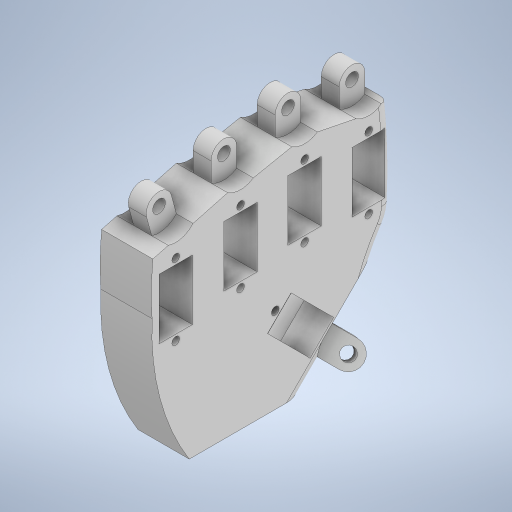
# Autodesk Inventor part: 손바닥
Saved by Autodesk Inventor 2024 (Build 280153000, 153)
## iProperties
Created: 2023-05-04
Part Number: 손바닥
Material: 일반
Document SubType Name: Modeling
Designer: Lenovo
Density: 1 g/cm^3
Appearance: 기본값
Author: Lenovo
Autodesk Inventor part; units mm, degrees
sketch "스케치1" plane through (0, 0, 0) normal (1, 0, 0) x (0, 1, 0)
  circle A0 centre (0, 0) radius 2.5
  arc A1 (0, -5) -> (0, 5) centre (0, 0) ccw
  arc A2 (-7.4833, 5) -> (-7.4833, -5) centre (0, 0) ccw
  line L0 (0, 5) -> (-7.4833, 5)
  line L1 (0, -5) -> (-7.4833, -5)
  line L2 (-7.4833, 5) -> (-7.4833, 20)
  circle A3 centre (3, 25) radius 2.5
  arc A4 (3, 20) -> (3, 30) centre (3, 25) ccw
  arc A5 (-4.4833, 30) -> (-4.4833, 20) centre (3, 25) ccw
  line L3 (3, 30) -> (-4.4833, 30)
  line L4 (3, 20) -> (-4.4833, 20)
  line L5 (-7.4833, 20) -> (-4.4833, 20)
  circle A6 centre (0, 50) radius 2.5
  arc A7 (0, 45) -> (0, 55) centre (0, 50) ccw
  arc A8 (-7.4833, 55) -> (-7.4833, 45) centre (0, 50) ccw
  line L6 (0, 55) -> (-7.4833, 55)
  line L7 (0, 45) -> (-7.4833, 45)
  line L8 (-4.4833, 30) -> (-7.4833, 30)
  line L9 (-7.4833, 30) -> (-7.4833, 45)
  line L10 (-7.4833, 55) -> (-11.1068, 68.523)
  circle A9 centre (-5.1725, 75.2894) radius 2.5
  arc A10 (-3.8785, 70.4598) -> (-6.4666, 80.119) centre (-5.1725, 75.2894) ccw
  arc A11 (-13.695, 78.1822) -> (-11.1068, 68.523) centre (-5.1725, 75.2894) ccw
  line L11 (-6.4666, 80.119) -> (-13.695, 78.1822)
  line L12 (-3.8785, 70.4598) -> (-11.1068, 68.523)
  line L13 (-13.695, 78.1822) -> (-11.1068, 68.523) construction
  line L14 (-16.4833, 6.5) -> (-39.9833, 6.5)
  line L15 (-39.9833, 6.5) -> (-39.9833, -6.5)
  line L16 (-39.9833, -6.5) -> (-16.4833, -6.5)
  line L17 (-16.4833, -6.5) -> (-16.4833, 6.5)
  line L18 (-16.4833, 6.5) -> (-39.9833, -6.5) construction
  line L19 (-39.9833, 6.5) -> (-16.4833, -6.5) construction
  line L20 (-13.4833, 31.5) -> (-36.9833, 31.5)
  line L21 (-36.9833, 31.5) -> (-36.9833, 18.5)
  line L22 (-36.9833, 18.5) -> (-13.4833, 18.5)
  line L23 (-13.4833, 18.5) -> (-13.4833, 31.5)
  line L24 (-13.4833, 31.5) -> (-36.9833, 18.5) construction
  line L25 (-36.9833, 31.5) -> (-13.4833, 18.5) construction
  line L26 (-6.4666, 80.119) -> (-3.8785, 70.4598)
  line L27 (-0.3429, 76.5835) -> (-10.0022, 73.9953)
  line L28 (-16.8333, 6.2) -> (-39.6333, 6.2) construction
  line L29 (-39.6333, 6.2) -> (-39.6333, -6.2) construction
  line L30 (-39.6333, -6.2) -> (-16.8333, -6.2) construction
  line L31 (-16.8333, -6.2) -> (-16.8333, 6.2) construction
  line L32 (-39.6333, 6.2) -> (-16.8333, -6.2) construction
  line L33 (-16.8333, 6.2) -> (-39.6333, -6.2) construction
  circle A12 centre (-14.2333, 0) radius 1.5
  circle A13 centre (-42.2333, 0) radius 1.5
  circle A14 centre (-11.2333, 25) radius 1.5
  circle A15 centre (-39.2333, 25) radius 1.5
  line L34 (-11.2333, 25) -> (-13.4833, 25) construction
  line L35 (-39.2333, 25) -> (-36.9833, 25) construction
  line L36 (-7.4833, -5) -> (-8.9833, -9)
  arc A16 (-7.4833, 45) -> (-4.4833, 30) centre (31.5167, 45) ccw
  arc A17 (-4.4833, 20) -> (-7.4833, 5) centre (31.5167, 5) ccw
  line L37 (-15.6926, 45.7419) -> (-11.3799, 46.3097) construction
  line L38 (-11.3799, 46.3097) -> (-12.8345, 57.3589) construction
  line L39 (-13.695, 78.1822) -> (-15.3027, 84.1822)
  arc A18 (-15.3027, 84.1822) -> (-35.3027, 84.5) centre (-27.2025, -35.2263) ccw
  arc A19 (-35.3027, 84.5) -> (-90, 70) centre (-39.4128, -10.411) ccw
  arc A20 (-42.4833, -10) -> (-8.9833, -9) centre (-31.6798, 189.708) ccw
  line L40 (-90, 70) -> (-90, 15)
  line L41 (-90, 15) -> (-77.9792, 2.9792)
  arc A21 (-49.9792, -7.5208) -> (-42.4833, -10) centre (-41.6703, 5.0299) ccw
  arc A22 (-49.9792, -7.5208) -> (-77.9792, 2.9792) centre (-86.8108, -63.1552) ccw
  line L42 (-16.4833, 56.5) -> (-39.9833, 56.5)
  line L43 (-39.9833, 43.5) -> (-16.4833, 43.5)
  line L44 (-39.9833, 56.5) -> (-39.9833, 43.5)
  line L45 (-16.4833, 43.5) -> (-16.4833, 56.5)
  line L46 (-16.4833, 56.5) -> (-39.9833, 43.5) construction
  line L47 (-39.9833, 56.5) -> (-16.4833, 43.5) construction
  circle A23 centre (-42.2333, 50) radius 1.5
  circle A24 centre (-14.2333, 50) radius 1.5
  line L48 (-14.2333, 50) -> (-16.4833, 50) construction
  line L49 (-42.2333, 50) -> (-39.9833, 50) construction
  line L50 (-21.6555, 81.7894) -> (-45.1555, 81.7894)
  line L51 (-45.1555, 68.7894) -> (-21.6555, 68.7894)
  line L52 (-45.1555, 81.7894) -> (-45.1555, 68.7894)
  line L53 (-21.6555, 68.7894) -> (-21.6555, 81.7894)
  line L54 (-21.6555, 81.7894) -> (-45.1555, 68.7894) construction
  line L55 (-45.1555, 81.7894) -> (-21.6555, 68.7894) construction
  circle A25 centre (-47.4055, 75.2894) radius 1.5
  circle A26 centre (-19.4055, 75.2894) radius 1.5
  line L56 (-19.4055, 75.2894) -> (-21.6555, 75.2894) construction
  line L57 (-47.4055, 75.2894) -> (-45.1555, 75.2894) construction
  line L58 (-7.4833, 5) -> (-4.4833, 20)
  line L59 (-4.4833, 30) -> (-7.4833, 45)
  line L60 (-21.6555, 68.7894) -> (-16.7555, 68.7894)
  line L61 (-16.7555, 68.7894) -> (-16.7555, 81.7894)
  line L62 (-16.7555, 81.7894) -> (-21.6555, 81.7894)
  point P0 (-28.2333, 0)
  point P1 (-25.2333, 25)
  point P2 (-25.2333, 25)
  point P3 (-28.2333, 0)
  point P4 (-28.2333, 0)
  point P5 (-28.2333, 50)
  point P6 (-28.2333, 50)
  point P7 (-33.4055, 75.2894)
  point P8 (-33.4055, 75.2894)
  dimension "d0" = 5
  dimension "d1" = 10
  dimension "d2" = 18
  dimension "d3" = 15
  dimension "d4" = 5
  dimension "d5" = 10
  dimension "d6" = 18
  dimension "d8" = 3
  dimension "d9" = 5
  dimension "d10" = 10
  dimension "d11" = 18
  dimension "d13" = 15
  dimension "d14" = 3
  dimension "d15" = 14
  dimension "d16" = 165
  dimension "d17" = 5
  dimension "d18" = 10
  dimension "d19" = 18
  dimension "d21" = 13
  dimension "d22" = 23.5
  dimension "d24" = 13
  dimension "d25" = 23.5
  dimension "d26" = 9
  dimension "d33" = 9
  dimension "d34" = 22.8
  dimension "d35" = 12.4
  dimension "d36" = 3
  dimension "d37" = 2.6
  dimension "d38" = 3
  dimension "d39" = 2.6
  dimension "d40" = 3
  dimension "d41" = 3
  dimension "d44" = 28
  dimension "d56" = 90
  dimension "d57" = 70
  dimension "d82" = 6
  dimension "d83" = 20
  dimension "d84" = 120
  dimension "d85" = 95
  dimension "d86" = 84.5
  dimension "d94" = 1.5
  dimension "d95" = 35
  dimension "d96" = 200
  dimension "d97" = 4
  dimension "d98" = 5
  dimension "d100" = 25
  dimension "d107" = 17
  dimension "d108" = 135
  dimension "d110" = 55
  dimension "d111" = 28
  dimension "d112" = 10.5
  dimension "d185" = 13
  dimension "d186" = 23.5
  dimension "d187" = 3
  dimension "d188" = 3
  dimension "d189" = 28
  dimension "d190" = 9
  dimension "d191" = 13
  dimension "d192" = 23.5
  dimension "d193" = 3
  dimension "d194" = 3
  dimension "d195" = 28
  dimension "d198" = 4.9
  dimension "d199" = 11.583
  constraints: 126 end point, 31 point on circle, 27 centre point, 18 midpoint, 14 parallel, 12 coincident, 12 horizontal alignment, 12 tangent, 11 horizontal, 10 perpendicular, 5 collinear, 2 vertical
  measures "d0" diameter of A0
  measures "d1" diameter of A1
  measures "d2" diameter of A2
  measures "d3" distance of L0.end L2.end
  measures "d4" diameter of A3
  measures "d5" diameter of A4
  measures "d6" diameter of A5
  measures "d8" distance of L2.end L4.end
  measures "d9" diameter of A6
  measures "d10" diameter of A7
  measures "d11" diameter of A8
  measures "d13" distance of L8.end L7.end
  measures "d14" distance of L3.end L8.end
  measures "d15" distance of L6.end L10.end
  measures "d16" angle of L9 L10
  measures "d17" diameter of A9
  measures "d18" diameter of A10
  measures "d19" diameter of A11
  measures "d21" distance of L16.end L14.start
  measures "d22" distance of L15.end L16.end
  measures "d24" distance of L22.end L20.start
  measures "d25" distance of L22.start L22.end
  measures "d26" distance from line of L4.end L23
  measures "d33" distance from line of L17 L1.end
  measures "d34" distance of L29.end L30.end
  measures "d35" distance of L28.end L29.end
  measures "d36" diameter of A12
  measures "d37" distance from line of L31 A12.centre
  measures "d38" diameter of A13
  measures "d39" distance from line of A13.centre L29
  measures "d40" diameter of A14
  measures "d41" diameter of A15
  measures "d44" distance of L35.start L34.start
  measures "d56" horizontal distance of point (0, 0) L40.start
  measures "d57" vertical distance of point (0, 0) L40.start
  measures "d82" vertical distance of L11.end L39.end
  measures "d83" horizontal distance of A18.end L39.end
  measures "d84" radius of A18
  measures "d85" radius of A19
  measures "d86" vertical distance of point (0, 0) A18.end
  measures "d94" horizontal distance of L36.end L1.end
  measures "d95" horizontal distance of A20.start L1.end
  measures "d96" radius of A20
  measures "d97" vertical distance of L36.end L1.end
  measures "d98" vertical distance of A20.start L1.end
  measures "d100" vertical distance of A20.start L40.end
  measures "d107" distance of L40.end L41.end
  measures "d108" angle of L41 L40
  measures "d110" distance of L40.start L40.end
  measures "d111" horizontal distance of L41.end A21.start
  measures "d112" vertical distance of L41.end A21.start
  measures "d185" distance of L47.end L42.start
  measures "d186" distance of L44.end L47.end
  measures "d187" diameter of A24
  measures "d188" diameter of A23
  measures "d189" distance of L49.start L48.start
  measures "d190" distance from line of L45 L7.end
  measures "d191" distance of L51.end L54.start
  measures "d192" distance of L52.end L51.end
  measures "d193" diameter of A26
  measures "d194" diameter of A25
  measures "d195" distance of L57.start L56.start
  measures "d198" distance of L51.end L60.end
  measures "d199" distance from line of A9.centre L61
extrude "돌출1" add sketch "스케치1" along normal mid plane 7 contours L1 A2 L0 A1 | A5 L3 A4 L4 | A8 L6 A7 L7 | A11 L11 L26 A9 L12 | L26 A9 L27 A10 | A10 L27 A9 L26
extrude "돌출2" add sketch "스케치1" along normal mid plane 20 contours L36 A20 A21 A22 L41 L40 A19 A18 L39 A11 L10 A8 L9 L8 A5 L5 L2 A2 | L2 L5 A17 | A17 L58 | L8 L9 A16 | A16 L59 | L62 L61 L60 L53
sketch "스케치2" plane through (-10, 0, 0) normal (1, 0, 0) x (0, 0, -1)
  line L0 (-31.5, -36.9833) -> (-31.5, -13.4833) projected
  line L1 (-18.5, -13.4833) -> (-18.5, -36.9833) projected
  line L2 (-6.5, -39.9833) -> (-6.5, -16.4833) projected
  line L3 (6.5, -16.4833) -> (6.5, -39.9833) projected
  line L4 (-31.5, -13.4833) -> (-18.5, -13.4833) projected
  line L5 (-31.5, -13.4833) -> (-31.5, -8.5833)
  line L6 (-31.5, -8.5833) -> (-18.5, -8.5833)
  line L7 (-18.5, -8.5833) -> (-18.5, -13.4833)
  line L8 (-31.5, -36.9833) -> (-31.5, -41.8833)
  line L9 (-31.5, -41.8833) -> (-18.5, -41.8833)
  line L10 (-18.5, -41.8833) -> (-18.5, -36.9833)
  line L11 (-6.5, -39.9833) -> (-6.5, -44.8833)
  line L12 (-6.5, -44.8833) -> (6.5, -44.8833)
  line L13 (6.5, -44.8833) -> (6.5, -39.9833)
  line L14 (-6.5, -16.4833) -> (6.5, -16.4833) projected
  line L15 (-6.5, -16.4833) -> (-6.5, -11.5833)
  line L16 (-6.5, -11.5833) -> (6.5, -11.5833)
  line L17 (6.5, -11.5833) -> (6.5, -16.4833)
  line L18 (-43.5, -39.9833) -> (-43.5, -16.4833) projected
  line L19 (-43.5, -16.4833) -> (-56.5, -16.4833) projected
  line L20 (-56.5, -16.4833) -> (-56.5, -39.9833) projected
  line L21 (-56.5, -39.9833) -> (-43.5, -39.9833) projected
  line L22 (-43.5, -16.4833) -> (-43.5, -11.5833)
  line L23 (-43.5, -11.5833) -> (-56.5, -11.5833)
  line L24 (-56.5, -11.5833) -> (-56.5, -16.4833)
  line L25 (-43.5, -39.9833) -> (-43.5, -44.8833)
  line L26 (-43.5, -44.8833) -> (-56.5, -44.8833)
  line L27 (-56.5, -44.8833) -> (-56.5, -39.9833)
  line L28 (-68.7894, -45.1555) -> (-68.7894, -21.6555) projected
  line L29 (-68.7894, -21.6555) -> (-81.7894, -21.6555) projected
  line L30 (-81.7894, -21.6555) -> (-81.7894, -45.1555) projected
  line L31 (-81.7894, -45.1555) -> (-68.7894, -45.1555) projected
  line L32 (-68.7894, -21.6555) -> (-68.7894, -16.7555)
  line L33 (-68.7894, -16.7555) -> (-81.7894, -16.7555)
  line L34 (-81.7894, -16.7555) -> (-81.7894, -21.6555)
  line L35 (-68.7894, -45.1555) -> (-68.7894, -50.0555)
  line L36 (-68.7894, -50.0555) -> (-81.7894, -50.0555)
  line L37 (-81.7894, -50.0555) -> (-81.7894, -45.1555)
  point P0 (0, 0)
  dimension "d67" = 4.9
  dimension "d68" = 4.9
  dimension "d69" = 4.9
  dimension "d70" = 4.9
  dimension "d196" = 4.9
  dimension "d197" = 4.9
  dimension "d200" = 4.9
  dimension "d201" = 4.9
  constraints: 48 end point, 13 perpendicular, 7 vertical, 4 point on line, 3 parallel, 1 collinear
  measures "d67" distance of L0.end L5.end
  measures "d68" distance of L0.start L8.end
  measures "d69" distance of L2.start L11.end
  measures "d70" distance of L2.end L15.end
  measures "d196" distance of L26.end L20.end
  measures "d197" distance of L23.end L19.end
  measures "d200" distance of L33.end L29.end
  measures "d201" distance of L36.end L30.end
extrude "돌출3" cut sketch "스케치2" along normal blind 4 contours L0 L4 L1 L10 L9 L8 | L5 L6 L7 L4 | L2 L14 L3 L13 L12 L11 | L15 L16 L17 L14 | L25 L26 L27 L21 | L19 L24 L23 L22 | L35 L36 L37 L31 | L29 L34 L33 L32
sketch "스케치3" plane through (10, 0, 0) normal (1, 0, 0) x (0, 0, -1)
  line L0 (-70, -90) -> (-15, -90) projected
  line L1 (-15, -90) -> (8.5931, -66.4069)
  line L2 (-97.2929, 0) -> (55.0772, 0) construction
  line L3 (0, 13.6483) -> (0, -114.1231) construction
  point P0 (0, 0)
  dimension "d102" = 45
  constraints: 6 end point, 1 horizontal, 1 horizontal alignment, 1 vertical, 1 vertical alignment
  measures "d102" angle of L1 L3
ref_plane "작업 평면2" through (10, -90, 15) normal (0.7071068, -0.5, -0.5) x (0, 0.7071068, -0.7071068)
ref_plane "작업 평면4" through (0, -90, 15) normal (-0.7071068, -0.5, -0.5) x (0, 0.7071068, -0.7071068)
sketch "스케치4" plane through (0, -90, 15) normal (-0.7071068, -0.5, -0.5) x (0, 0.7071068, -0.7071068)
  circle A0 centre (8.5, 8) radius 5
  line L0 (-114.8654, 0) -> (162.4605, 0) projected
  line L1 (3.5, 8) -> (3.5, 0)
  line L2 (13.5, 8) -> (13.5, 0)
  line L3 (0, 7.0711) -> (17, 7.0711) projected
  line L4 (8.5, 13.003) -> (8.5, -11.2228) construction
  circle A1 centre (8.5, 8) radius 9
  circle A2 centre (8.5, 8) radius 2.5
  line L5 (3.5, 0) -> (3.5, -4)
  line L6 (3.5, -4) -> (13.5, -4)
  line L7 (13.5, -4) -> (13.5, 0)
  point P0 (74.2462, -37.5)
  point P1 (8.5, 7.0711)
  point P2 (13.5, 7.0711)
  point P3 (13.413, 7.0711)
  point P4 (3.587, 7.0711)
  point P5 (3.5, 7.0711)
  dimension "d114" = 10
  dimension "d115" = 18
  dimension "d116" = 8
  dimension "d117" = 5
  dimension "d118" = 4
  constraints: 12 end point, 4 perpendicular, 3 centre point, 2 coincident, 2 point on circle, 2 point on line, 2 tangent, 2 vertical, 2 vertical alignment, 1 midpoint
  measures "d114" diameter of A0
  measures "d115" diameter of A1
  measures "d116" distance from line of L0 A1.centre
  measures "d117" diameter of A2
  measures "d118" distance of L6.end L2.end
chamfer "모따기1" distance 10 angle 45 1 edges at (10, -83.9896, 8.9896)
ref_plane "작업 평면5" through (5, -90, 22.0711) normal (-0.7068323, -0.480107, -0.5195049) x (0.019699, 0.7207616, -0.6929031)
sketch "스케치5" plane through (5, -90, 22.0711) normal (-0.7068323, -0.480107, -0.5195049) x (0.019699, 0.7207616, -0.6929031)
  arc A0 (18.2978, 0.0167) -> (18.2727, 0) centre (13.2978, 7.5) ccw
  circle A1 centre (13.2978, 7.5) radius 5
  circle A2 centre (13.2978, 7.5) radius 2.5
  line L0 (4.8011, 0) -> (21.7945, 0) projected
  line L1 (8.2978, 7.5) -> (8.2978, 0)
  line L2 (18.2978, 7.5) -> (18.2978, 0)
  line L3 (8.2978, 0) -> (18.2978, 0.0167)
  line L4 (50.6015, -1.5) -> (2.0363, -1.5)
  line L5 (50.6015, -1.5) -> (50.6015, 2.5)
  line L6 (50.6015, 2.5) -> (20.7811, 2.5)
  line L7 (18.2978, 0.0167) -> (18.2978, -1.5)
  point P0 (80.0632, -37.5)
  point P1 (18.2958, 0)
  point P2 (13.2978, 0)
  point P3 (8.3228, 0)
  point P4 (13.2978, -1.5)
  point P5 (18.2978, 0)
  dimension "d145" = 18
  dimension "d146" = 10
  dimension "d147" = 5
  dimension "d148" = 7.5
  constraints: 14 end point, 6 point on line, 5 point on circle, 3 centre point, 3 tangent, 2 coincident, 2 perpendicular, 1 horizontal, 1 midpoint, 1 parallel, 1 vertical, 1 vertical alignment
  measures "d145" diameter of A0
  measures "d146" diameter of A1
  measures "d147" diameter of A2
  measures "d148" distance of L1.start L1.end
extrude "돌출10" cut sketch "스케치5" along normal mid plane 100 contours A0 L6 L5 L4 L7 L2 | L7 L4 A0 L0 | L0 A0
extrude "돌출9" add sketch "스케치5" along normal mid plane 7 contours L3 A0 L1 A1 L2 | L2 L0 L3 | A1 | L7 L4 A0 L0 | L0 L1 A0 | L0 A0
fillet "모깎기3" radius 5 3 edges at (10, -25.7123, -10.203) (10, -50.4875, -7.1876) (10, -46.3967, -9.2606)
fillet "모깎기4" radius 3 3 edges at (-10, -46.3967, -9.2606) (-10, -63.3834, -0.6819) (-10, -25.7123, -10.203)
fillet "모깎기5" radius 5 2 edges at (10, -85.3582, 24.5003) (0, -88.7544, 13.7544)
sketch "스케치7" plane through (-10, 0, 0) normal (-1, 0, 0) x (0, 0, 1)
  line L0 (22.8559, -79.4711) -> (39.4729, -62.8541)
  line L1 (39.4729, -62.8541) -> (30.2805, -53.6617)
  line L2 (30.2805, -53.6617) -> (13.6635, -70.2787)
  line L3 (13.6635, -70.2787) -> (22.8559, -79.4711)
  line L4 (22.8559, -79.4711) -> (30.2805, -53.6617) construction
  line L5 (39.4729, -62.8541) -> (13.6635, -70.2787) construction
  line L6 (22.8912, -79.0115) -> (39.0133, -62.8894) construction
  line L7 (39.0133, -62.8894) -> (30.2451, -54.1213) construction
  line L8 (30.2451, -54.1213) -> (14.1231, -70.2434) construction
  line L9 (14.1231, -70.2434) -> (22.8912, -79.0115) construction
  line L10 (39.0133, -62.8894) -> (14.1231, -70.2434) construction
  line L11 (22.8912, -79.0115) -> (30.2451, -54.1213) construction
  circle A0 centre (16.6687, -76.4659) radius 1.5
  circle A1 centre (36.4677, -56.6669) radius 1.5
  line L12 (6.3523, -81.3523) -> (15, -90) projected
  line L13 (16.6687, -76.4659) -> (18.2597, -74.8749) construction
  line L14 (36.4677, -56.6669) -> (34.8767, -58.2579) construction
  ellipse E0 centre (7.2887, -85.8459) end of major axis (8.9855, -87.6819) minor radius 1.7671 projected
  line L15 (7.2887, -85.8459) -> (38.3363, -54.7983)
  circle A2 centre (-4.1034, -102.3354) radius 25.5
  point P0 (0, 0)
  point P1 (22.3195, -70.4311)
  point P2 (22.3195, -70.4311)
  point P3 (22.3195, -70.4311)
  point P4 (22.4093, -66.6452)
  point P5 (8.8825, -65.4012)
  dimension "d158" = 13
  dimension "d159" = 23.5
  dimension "d160" = 22.8
  dimension "d161" = 12.4
  dimension "d162" = 3
  dimension "d163" = 2.6
  dimension "d164" = 3
  dimension "d165" = 2.6
  dimension "d167" = 13
  dimension "d181" = 51
  dimension "d182" = 0.3
  dimension "d183" = 0.35
  dimension "d184" = 0
  constraints: 30 end point, 4 parallel, 4 perpendicular, 3 centre point, 2 midpoint, 1 collinear
  measures "d158" distance of L3.start L3.end
  measures "d159" distance of L4.end L3.start
  measures "d160" distance of L11.end L9.start
  measures "d161" distance of L6.end L11.end
  measures "d162" diameter of A0
  measures "d163" distance from line of L9 L13.start
  measures "d164" diameter of A1
  measures "d165" distance from line of L14.start L7
  measures "d167" distance between parallel lines of L3 L12
  measures "d181" diameter of A2
  measures "d182" distance between parallel lines of L2 L8
  measures "d183" distance between parallel lines of L9 L3
  measures "d184" distance from line of L15 L13.start
extrude "돌출11" cut sketch "스케치7" against normal blind 29 contours L3 L15 L1 L0 | L3 L2 L1 L15 | A1 L15 | L15 A1
extrude "돌출12" cut sketch "스케치7" against normal blind 13 contours A0 L15 | L15 A0
sketch "스케치8" plane through (-10, 0, 0) normal (-1, 0, 0) x (0, 0, 1)
  line L0 (22.8559, -79.4711) -> (13.6635, -70.2787) projected
  line L1 (39.4729, -62.8541) -> (22.8559, -79.4711) projected
  line L2 (30.2805, -53.6617) -> (39.4729, -62.8541) projected
  line L3 (13.6635, -70.2787) -> (30.2805, -53.6617) projected
  line L4 (13.6635, -70.2787) -> (10.1987, -73.7435)
  line L5 (10.1987, -73.7435) -> (19.3911, -82.9359)
  line L6 (19.3911, -82.9359) -> (22.8559, -79.4711)
  line L7 (39.4729, -62.8541) -> (42.9377, -59.3893)
  line L8 (42.9377, -59.3893) -> (33.7453, -50.1969)
  line L9 (33.7453, -50.1969) -> (30.2805, -53.6617)
  point P0 (0, 0)
  dimension "d177" = 4.9
  dimension "d178" = 4.9
  constraints: 12 end point, 4 perpendicular, 3 point on line
  measures "d177" distance of L8.end L2.start
  measures "d178" distance of L0.end L4.end
extrude "돌출13" cut sketch "스케치8" against normal blind 8.5 contours L6 L5 L4 L0 | L2 L9 L8 L7
